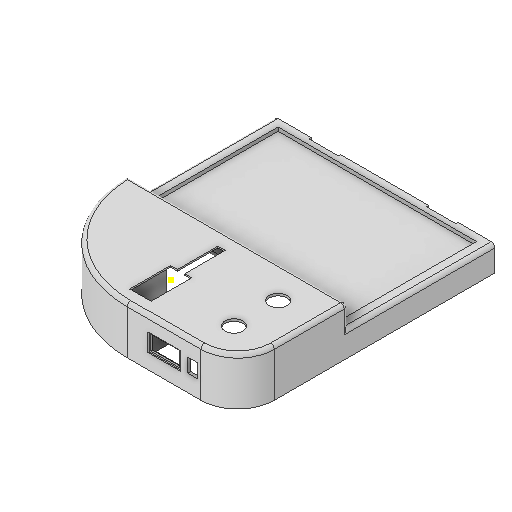
# Autodesk Inventor part: PLATE 1
Saved by Autodesk Inventor 2025.3 (Build 293356030, 356C)
## iProperties
Created: 2025-09-25
Part Number: PLATE 1
Material: 일반
Document SubType Name: Modeling
Designer: joseph
Density: 1 g/cm^3
Appearance: 기본값
Mass: 533.124 g
Surface Area: 3433.78 cm^2
Volume: 533.124 cm^3
Author: joseph
Autodesk Inventor part; units mm, degrees
ref_plane "YZ Plane" through (0, 0, 0) normal (1, 0, 0) x (0, 1, 0)
ref_plane "XZ Plane" through (0, 0, 0) normal (0, 1, 0) x (-1, 0, 0)
ref_plane "XY Plane" through (0, 0, 0) normal (0, 0, 1) x (1, 0, 0)
sketch "스케치6" plane through (0, 0, 0) normal (0, 0, 1) x (1, 0, 0)
  circle A0 centre (0, 0) radius 50
  line L0 (150, 90) -> (-150, 90)
  line L1 (-150, 90) -> (-150, 290)
  line L2 (-150, 290) -> (150, 290)
  line L3 (150, 290) -> (150, 90)
  line L4 (150, 90) -> (150, 14.5116)
  line L5 (0, -60) -> (100, -60)
  line L6 (150, 14.5116) -> (150, -10)
  arc A1 (-150, 90) -> (0, -60) centre (0, 90) ccw
  arc A2 (100, -60) -> (150, -10) centre (100, -10) ccw
  arc A3 (-147, 86) -> (17.5784, -56) centre (0, 90) ccw
  line L7 (17.5784, -56) -> (100, -56)
  arc A4 (100, -56) -> (146, -10) centre (100, -10) ccw
  line L8 (146, -10) -> (146, 14.5116)
  line L9 (146, 14.5116) -> (146, 86)
  line L10 (146, 86) -> (-147, 86)
  line L11 (-149.9467, 86) -> (-150, 86)
  point P0 (150, -60)
  point P1 (150, -60)
  point P2 (0, 290)
  dimension "d0" = 100
  dimension "d1" = 300
  dimension "d2" = 200
  dimension "d5" = 150
  dimension "d8" = 90
  dimension "d9" = 150
  dimension "d10" = 50
  dimension "d24" = 3
  constraints: 24 end point, 9 point on circle, 5 centre point, 4 parallel, 4 tangent, 3 point on line, 2 horizontal, 2 vertical, 1 coincident, 1 midpoint, 1 perpendicular, 1 vertical alignment, 2 other
  measures "d0" diameter of A0
  measures "d1" distance of L1.end L2.end
  measures "d2" distance of L0.end L1.end
  measures "d5" distance of L0.start point (150, -60)
  measures "d8" vertical distance of point (0, 0) L0.end
  measures "d9" distance of L5.start point (150, -60)
  measures "d10" radius of A2
  measures "d24" horizontal distance of L0.end L10.end
extrude "돌출1" add sketch "스케치6" against normal blind 65 contours L4 L6 A2 L5 A1 L0
extrude "돌출2" add sketch "스케치6" against normal blind 3 contours L10 L9 L8 A4 L7 A3
sketch "스케치8" plane through (-147, 86, -65) normal (0, -1, 0) x (1, 0, 0)
  line L0 (293, 62) -> (0, 62) projected
  line L1 (0, 62) -> (0, 0) projected
  line L2 (293, 0) -> (0, 0) projected
  line L3 (293, 62) -> (293, 0) projected
  line L4 (0, 0) -> (293, 0)
  line L5 (293, 0) -> (293, 27.5)
  line L6 (293, 27.5) -> (0, 27.5)
  line L7 (0, 27.5) -> (0, 0)
  point P0 (147, 65)
  dimension "d17" = 27.5
  constraints: 8 end point, 2 parallel, 1 horizontal, 1 perpendicular, 1 point on line
  measures "d17" distance of L5.end L4.end
extrude "돌출3" cut sketch "스케치8" against normal blind 60 contours L3 L2 L1 L6
sketch "스케치9" plane through (0, 0, -65) normal (0, 0, -1) x (-1, 0, 0)
  line L0 (-146, -10) -> (-146, 90) projected
  line L1 (-146, 90) -> (-150, 90) projected
  line L2 (-150, 90) -> (-150, -10) projected
  arc A0 (-150, -10) -> (-100, -60) centre (-100, -10) ccw projected
  line L3 (-100, -60) -> (0, -60) projected
  arc A1 (0, -60) -> (150, 90) centre (0, 90) ccw projected
  line L4 (150, 90) -> (147, 90) projected
  line L5 (147, 90) -> (147, 86) projected
  arc A2 (-17.5784, -56) -> (147, 86) centre (0, 90) ccw projected
  line L6 (-17.5784, -56) -> (-100, -56) projected
  arc A3 (-146, -10) -> (-100, -56) centre (-100, -10) ccw projected
  line L7 (-150, 90) -> (150, 90)
  line L8 (150, 90) -> (150, 290)
  line L9 (150, 290) -> (-150, 290)
  line L10 (-150, 290) -> (-150, 90)
  line L11 (-146, 90) -> (146, 90)
  line L12 (146, 90) -> (146, 286)
  line L13 (146, 286) -> (-146, 286)
  line L14 (-146, 286) -> (-146, 90)
  point P0 (0, 0)
  point P1 (146, 90)
  dimension "d20" = 300
  dimension "d21" = 200
  dimension "d22" = 292
  dimension "d23" = 196
  constraints: 16 end point, 4 parallel, 2 horizontal, 2 perpendicular
  measures "d20" distance of L9.end L8.end
  measures "d21" distance of L8.end L7.end
  measures "d22" distance of L13.end L12.end
  measures "d23" distance of L12.end L11.end
extrude "돌출4" add sketch "스케치9" against normal blind 34.5 contours L1 L10 L9 L8 L4 L7 L12 L13 L14
sketch "스케치10" plane through (0, 0, -30.5) normal (0, 0, 1) x (1, 0, 0)
  line L0 (150, 290) -> (-150, 290) projected
  line L1 (-150, 290) -> (-150, 90) projected
  line L2 (-146, 90) -> (-150, 90) projected
  line L3 (-146, 90) -> (-146, 286) projected
  line L4 (-146, 286) -> (146, 286) projected
  line L5 (146, 286) -> (146, 90) projected
  line L6 (150, 90) -> (146, 90) projected
  line L7 (150, 90) -> (150, 290) projected
  line L8 (-150, 90) -> (150, 90)
  point P0 (0, 0)
  point P1 (-146, 90)
  constraints: 2 end point, 1 horizontal
extrude "돌출5" add sketch "스케치10" against normal blind 7
fillet "모깎기1" radius 5 2 edges at (150, 190, -30.5) (-150, 190, -30.5)
fillet "모깎기2" radius 5 7 edges at (150, 90, -33) (150, 90, -15.25) (135.3553, -45.3553, 0) (50, -60, 0) (-106.066, -16.066, 0) (150, 40, 0) (0, 90, 0)
sketch "스케치12" plane through (0, 0, 0) normal (0, 0, 1) x (1, 0, 0)
  circle A0 centre (100, -15) radius 22.5
  circle A1 centre (100, 45) radius 22.5
  circle A2 centre (100, 45) radius 12.15
  circle A3 centre (100, -15) radius 12.15
  point P0 (0, 0)
  dimension "d33" = 45
  dimension "d34" = 45
  dimension "d35" = 15
  dimension "d36" = 100
  dimension "d37" = 60
  dimension "d38" = 24.3
  dimension "d39" = 24.3
  constraints: 4 centre point, 2 coincident, 1 vertical alignment
  measures "d33" diameter of A0
  measures "d34" diameter of A1
  measures "d35" vertical distance of A0.centre point (0, 0)
  measures "d36" horizontal distance of A0.centre point (0, 0)
  measures "d37" distance of A0.centre A1.centre
  measures "d38" diameter of A2
  measures "d39" diameter of A3
extrude "돌출6" cut sketch "스케치12" against normal through all contours A2 | A3
sketch "스케치13" plane through (0, 0, -65) normal (0, 0, -1) x (-1, 0, 0)
  line L0 (-150, 290) -> (-150, -10) projected
  arc A0 (-150, -10) -> (-100, -60) centre (-100, -10) ccw projected
  line L1 (-100, -60) -> (0, -60) projected
  arc A1 (0, -60) -> (150, 90) centre (0, 90) ccw projected
  line L2 (150, 90) -> (150, 290) projected
  line L3 (150, 290) -> (-150, 290) projected
  line L4 (-146, -10) -> (-146, 286) projected
  line L5 (-146, 286) -> (146, 286) projected
  line L6 (147, 90) -> (147, 86) projected
  arc A2 (-17.5784, -56) -> (147, 86) centre (0, 90) ccw projected
  line L7 (-17.5784, -56) -> (-100, -56) projected
  arc A3 (-146, -10) -> (-100, -56) centre (-100, -10) ccw projected
  circle A4 centre (-100, -15) radius 12.15 projected
  line L8 (-100, -36) -> (-16.3347, -36)
  arc A5 (-16.3347, -36) -> (127, 86.282) centre (0, 90) ccw
  line L9 (127, 86.282) -> (127, 266)
  line L10 (127, 266) -> (-126, 266)
  line L11 (-126, 266) -> (-126, -10)
  arc A6 (-126, -10) -> (-100, -36) centre (-100, -10) ccw
  line L12 (146, 286) -> (146, 90) projected
  line L13 (146, 90) -> (147, 90) projected
  point P0 (0, 0)
  dimension "d42" = 20
  constraints: 8 end point, 4 point on circle, 2 centre point, 5 other
  measures "d42" radial gap between concentric circles of A3 A6
extrude "돌출7" add sketch "스케치13" against normal blind 3 contours L4 L5 L12 L13 L6 A2 L7 A3
sketch "스케치15" plane through (-150, 90, -65) normal (-1, 0, 0) x (0, 0, 1)
  line L0 (29.5, 200) -> (29.5, 0) projected
  line L1 (0, 200) -> (29.5, 200) projected
  line L2 (0, 0) -> (0, 200) projected
  line L3 (29.5, 0) -> (0, 0) projected
  line L4 (9.75, 190) -> (19.75, 190)
  line L5 (19.75, 190) -> (19.75, 195)
  line L6 (19.75, 195) -> (9.75, 195)
  line L7 (9.75, 195) -> (9.75, 190)
  point P0 (65, -90)
  point P1 (14.75, 195)
  point P2 (14.75, 200)
  dimension "d45" = 10
  dimension "d46" = 5
  dimension "d47" = 5
  constraints: 8 end point, 2 midpoint, 2 parallel, 1 horizontal, 1 perpendicular, 1 vertical alignment
  measures "d45" distance of L6.end L5.end
  measures "d46" distance of L5.end L4.end
  measures "d47" distance between parallel lines of L1 L6
extrude "돌출8" cut sketch "스케치15" against normal blind 10 contours L7 L6 L5 L4
sketch "스케치16" plane through (0, 0, -30.5) normal (0, 0, 1) x (1, 0, 0)
  line L0 (-145, 90) -> (-145, 290) projected
  line L1 (145, 90) -> (-145, 90) projected
  line L2 (145, 290) -> (145, 90) projected
  line L3 (145, 290) -> (-145, 290) projected
  line L4 (-135, 280) -> (-135, 100)
  line L5 (-135, 100) -> (135, 100)
  line L6 (135, 100) -> (135, 280)
  line L7 (135, 280) -> (-135, 280)
  point P0 (0, 0)
  dimension "d50" = 10
  constraints: 8 end point, 3 other
  measures "d50" distance between parallel lines of L0 L4
extrude "돌출9" cut sketch "스케치16" against normal blind 5 contours L7 L6 L5 L4
sketch "스케치17" plane through (0, 0, 0) normal (0, 0, 1) x (1, 0, 0)
  line L0 (-25, 13.2) -> (25, 13.2)
  line L1 (25, 13.2) -> (25, -55.3)
  line L2 (25, -55.3) -> (-25, -55.3)
  line L3 (-25, -55.3) -> (-25, 13.2)
  line L4 (-20.35, 13.2) -> (20.35, 13.2)
  line L5 (20.35, 13.2) -> (20.35, -48)
  line L6 (20.35, -48) -> (-20.35, -48)
  line L7 (-20.35, -48) -> (-20.35, 13.2)
  line L8 (-14.5, 13.2) -> (14.5, 13.2)
  line L9 (14.5, 13.2) -> (14.5, -42.2)
  line L10 (14.5, -42.2) -> (-14.5, -42.2)
  line L11 (-14.5, -42.2) -> (-14.5, 13.2)
  line L12 (-25, -51.9991) -> (0, -55.3)
  point P0 (0, 0)
  point P1 (0, -48)
  point P2 (0, -42.2)
  point P3 (-14.5, 13.2)
  point P4 (0, 13.2)
  dimension "d53" = 50
  dimension "d54" = 68.5
  dimension "d55" = 13.2
  dimension "d56" = 40.7
  dimension "d57" = 61.2
  dimension "d58" = 29
  dimension "d59" = 55.4
  constraints: 26 end point, 6 parallel, 4 midpoint, 3 horizontal, 3 perpendicular, 3 point on line, 3 vertical alignment
  measures "d53" distance of L1.end L2.end
  measures "d54" distance of L0.end L1.end
  measures "d55" distance from line of point (0, 0) L0
  measures "d56" distance of L5.end L6.end
  measures "d57" distance of L4.end L5.end
  measures "d58" distance of L9.end L10.end
  measures "d59" distance of L8.end L9.end
extrude "돌출10" add sketch "스케치17" against normal blind 2 contours L0 L7 L6 L5 L1 L2 L12 L3 | L0 L11 L10 L9 L5 L6 L7
sketch "스케치18" plane through (-25, 13.2, 0) normal (0, 1, 0) x (1, 0, 0)
  line L0 (10.5, 0) -> (0, 0) projected
  line L1 (10.5, 0) -> (10.5, 2) projected
  line L2 (0, 2) -> (10.5, 2) projected
  line L3 (0, 0) -> (0, 2) projected
  line L4 (50, 0) -> (39.5, 0) projected
  line L5 (50, 0) -> (50, 2) projected
  line L6 (39.5, 2) -> (50, 2) projected
  line L7 (39.5, 0) -> (39.5, 2) projected
  line L8 (50, 2) -> (0, 2)
  line L9 (0, 2) -> (0, 52)
  line L10 (0, 52) -> (50, 52)
  line L11 (50, 52) -> (50, 2)
  line L12 (39.5, 2) -> (45.2, 2)
  line L13 (45.2, 2) -> (45.2, 36.4)
  line L14 (45.2, 36.4) -> (39.5, 36.4)
  line L15 (39.5, 36.4) -> (39.5, 2)
  line L16 (10.5, 2) -> (4.8, 2)
  line L17 (4.8, 2) -> (4.8, 36.4)
  line L18 (4.8, 36.4) -> (10.5, 36.4)
  line L19 (10.5, 36.4) -> (10.5, 2)
  line L20 (10.5, 36.4) -> (4.8, 36.4)
  line L21 (4.8, 36.4) -> (4.8, 39.7)
  line L22 (4.8, 39.7) -> (10.5, 39.7)
  line L23 (10.5, 39.7) -> (10.5, 36.4)
  line L24 (45.2, 36.4) -> (39.5, 36.4)
  line L25 (39.5, 36.4) -> (39.5, 39.7)
  line L26 (39.5, 39.7) -> (45.2, 39.7)
  line L27 (45.2, 39.7) -> (45.2, 36.4)
  line L28 (39.5, 39.7) -> (10.5, 39.7)
  line L29 (10.5, 39.7) -> (10.5, 49.7)
  line L30 (10.5, 49.7) -> (39.5, 49.7)
  line L31 (39.5, 49.7) -> (39.5, 39.7)
  point P0 (25, 0)
  point P1 (0, 2)
  dimension "d62" = 50
  dimension "d63" = 5.7
  dimension "d64" = 34.4
  dimension "d65" = 5.7
  dimension "d66" = 34.4
  dimension "d67" = 3.3
  dimension "d68" = 10
  constraints: 48 end point, 12 parallel, 6 horizontal, 6 perpendicular, 4 point on line
  measures "d62" distance of L8.end L9.end
  measures "d63" distance of L14.end L13.end
  measures "d64" distance of L13.end L12.end
  measures "d65" distance of L17.end L18.end
  measures "d66" distance of L16.end L17.end
  measures "d67" distance of L20.end L21.end
  measures "d68" distance of L28.end L29.end
extrude "돌출11" add sketch "스케치18" against normal through all contours L9 L10 L11 L6 L13 L27 L26 L31 L30 L29 L22 L21 L17 L2 | L18 L21 L22 L23 | L25 L26 L27 L14
sketch "스케치19" plane through (0, 0, 0) normal (0, 0, 1) x (1, 0, 0)
  line L0 (100, -55) -> (25, -55) projected
  arc A0 (100, -55) -> (145, -10) centre (100, -10) ccw projected
  line L1 (145, 85) -> (145, -10) projected
  line L2 (-144.9138, 85) -> (145, 85) projected
  arc A1 (-144.9138, 85) -> (-2.4258, -54.9797) centre (0, 90) ccw projected
  line L3 (-2.4258, -54.9797) -> (0, -55.3) projected
  line L4 (0, -55.3) -> (25, -55.3) projected
  line L5 (25, -55.3) -> (25, -55) projected
  arc A2 (25, -43.3013) -> (-25, -43.3013) centre (0, 0) ccw projected
  line L6 (25, -43.3013) -> (25, 13.2) projected
  line L7 (25, 13.2) -> (14.5, 13.2) projected
  line L8 (14.5, 13.2) -> (14.5, -42.2) projected
  line L9 (14.5, -42.2) -> (-14.5, -42.2) projected
  line L10 (-14.5, -42.2) -> (-14.5, 13.2) projected
  line L11 (-14.5, 13.2) -> (-25, 13.2) projected
  line L12 (-25, 13.2) -> (-25, -43.3013) projected
  circle A3 centre (100, -15) radius 12.15 projected
  circle A4 centre (100, 45) radius 12.15 projected
  line L13 (-25, 13.2) -> (25, 13.2)
  constraints: 2 end point, 1 collinear
extrude "돌출12" add sketch "스케치19" against normal blind 2 contours L6 L7 L13 L11 L12 A2
sketch "스케치20" plane through (0, 0, -3) normal (0, 0, -1) x (-1, 0, 0)
  point P0 (0, 0)
sketch "스케치21" plane through (0, 0, -3) normal (0, 0, -1) x (-1, 0, 0)
  line L0 (147, 86) -> (-146, 86) projected
  line L1 (-25, 13.2) -> (25, 13.2) projected
  line L2 (-25, 13.2) -> (27.4279, 13.2)
  line L3 (27.4279, 13.2) -> (27.4279, 86)
  line L4 (27.4279, 86) -> (-25, 86)
  line L5 (-25, 86) -> (-25, 13.2)
  point P0 (0, 0)
  point P1 (22.5721, 13.2)
  constraints: 8 end point, 2 parallel, 1 horizontal, 1 perpendicular, 1 point on line
extrude "돌출13" cut sketch "스케치21" against normal blind 1
sketch "스케치22" plane through (0, 0, 0) normal (0, 0, 1) x (1, 0, 0)
  line L0 (-14.5, 13.2) -> (14.5, 13.2) projected
  line L1 (-5, 13.2) -> (5, 13.2)
  line L2 (5, 13.2) -> (5, 68.2)
  line L3 (5, 68.2) -> (-5, 68.2)
  line L4 (-5, 68.2) -> (-5, 13.2)
  point P0 (0, 0)
  point P1 (0, 13.2)
  dimension "d75" = 10
  dimension "d76" = 55
  constraints: 8 end point, 2 midpoint, 2 parallel, 1 horizontal, 1 perpendicular, 1 point on line
  measures "d75" distance of L3.end L2.end
  measures "d76" distance of L2.end L1.end
extrude "돌출14" cut sketch "스케치22" against normal blind 3
sketch "스케치23" plane through (25, 13.2, -52) normal (0, 0, -1) x (-1, 0, 0)
  line L0 (7.4216, -69.2) -> (0, -69.2) projected
  arc A0 (7.4216, -69.2) -> (50, -68.1138) centre (25, 76.8) ccw projected
  line L1 (50, 0) -> (50, -68.1138) projected
  line L2 (0, 0) -> (50, 0) projected
  line L3 (0, 0) -> (0, -69.2) projected
  circle A1 centre (7.5, -9) radius 1.6
  circle A2 centre (7.5, -31.9) radius 1.6
  circle A3 centre (42.2, -9) radius 1.6
  circle A4 centre (42.2, -31.9) radius 1.6
  point P0 (25, -13.2)
  dimension "d79" = 3.2
  dimension "d80" = 7.5
  dimension "d81" = 9
  dimension "d84" = 22.9
  dimension "d87" = 34.7
  constraints: 4 centre point, 1 horizontal, 1 vertical, 6 other
  measures "d79" diameter of A1
  measures "d80" horizontal distance of A1.centre L2.start
  measures "d81" vertical distance of L2.start A1.centre
  measures "d84" distance of A1.centre A2.centre
  measures "d87" distance of A1.centre A3.centre
extrude "돌출15" cut sketch "스케치23" against normal blind 20 contours A1 | A2 | A3 | A4
fillet "모깎기4" radius 10 11 edges at (132.5269, -42.5269, -3) (62.5, -56, -3) (146, 38, -3) (146, 86, -20.25) (85.5, 86, -3) (146, 186, -37.5) (-0.5, 86, -37.5) (-87.214, 86, -3) (-111.1763, -6.254, -3) (-25, -15.0506, -2) (25, -15.0506, -2)
fillet "모깎기5" radius 3.5 8 edges at (132.5269, -42.5269, -62) (146, 138, -62) (58.7892, -56, -62) (-96.065, -21.3396, -62) (-146, 188, -62) (0, 286, -62) (-146.5, 90, -62) (-147, 88, -62)
sketch "스케치24" plane through (0, -60, -65) normal (0, -1, 0) x (1, 0, 0)
  line L0 (30, 42.7) -> (70, 42.7)
  line L1 (70, 42.7) -> (70, 22.3)
  line L2 (70, 22.3) -> (30, 22.3)
  line L3 (30, 22.3) -> (30, 42.7)
  line L4 (0, 65) -> (0, 0) construction
  line L5 (16.3347, 0) -> (-127, 0) projected
  line L6 (72, 44.7) -> (28, 44.7)
  line L7 (28, 44.7) -> (28, 20.3)
  line L8 (28, 20.3) -> (72, 20.3)
  line L9 (72, 20.3) -> (72, 44.7)
  line L10 (82, 23) -> (96, 23)
  line L11 (96, 23) -> (96, 42)
  line L12 (96, 42) -> (82, 42)
  line L13 (82, 42) -> (82, 23)
  point P0 (30, 32.5)
  point P1 (0, 32.5)
  point P2 (82, 32.5)
  point P3 (72, 32.5)
  dimension "d94" = 40
  dimension "d95" = 20.4
  dimension "d96" = 30
  dimension "d97" = 2
  dimension "d102" = 14
  dimension "d103" = 19
  dimension "d104" = 10
  constraints: 26 end point, 6 parallel, 4 midpoint, 3 perpendicular, 2 horizontal, 2 horizontal alignment, 1 point on line, 1 vertical, 3 other
  measures "d94" distance of L1.end L2.end
  measures "d95" distance of L0.end L1.end
  measures "d96" horizontal distance of point (0, 32.5) L0.start
  measures "d97" distance between parallel lines of L0 L6
  measures "d102" distance of L12.end L11.end
  measures "d103" distance of L11.end L10.end
  measures "d104" distance between parallel lines of L9 L13
extrude "돌출16" cut sketch "스케치24" against normal blind 1.5 contours L9 L8 L7 L6
extrude "돌출17" cut sketch "스케치24" against normal blind 4 contours L0 L1 L2 L3
extrude "돌출18" cut sketch "스케치24" against normal blind 4 contours L13 L12 L11 L10
sketch "스케치25" plane through (-150, 290, -65) normal (0, 1, 0) x (1, 0, 0)
  arc A0 (0, -29.5) -> (5, -34.5) centre (5, -29.5) ccw projected
  line L0 (295, -34.5) -> (5, -34.5) projected
  arc A1 (295, -34.5) -> (300, -29.5) centre (295, -29.5) ccw projected
  line L1 (300, 0) -> (300, -29.5) projected
  line L2 (0, 0) -> (300, 0) projected
  line L3 (0, 0) -> (0, -29.5) projected
  line L4 (250, -34.5) -> (210, -34.5)
  line L5 (210, -34.5) -> (210, -18.5)
  line L6 (210, -18.5) -> (250, -18.5)
  line L7 (250, -18.5) -> (250, -34.5)
  line L8 (90, -34.5) -> (50, -34.5)
  line L9 (50, -34.5) -> (50, -18.5)
  line L10 (50, -18.5) -> (90, -18.5)
  line L11 (90, -18.5) -> (90, -34.5)
  point P0 (150, -65)
  dimension "d107" = 40
  dimension "d108" = 16
  dimension "d109" = 40
  dimension "d110" = 16
  dimension "d111" = 50
  dimension "d112" = 50
  constraints: 16 end point, 4 parallel, 2 horizontal, 2 perpendicular, 2 point on line
  measures "d107" distance of L5.end L6.end
  measures "d108" distance of L4.end L5.end
  measures "d109" distance of L9.end L10.end
  measures "d110" distance of L8.end L9.end
  measures "d111" distance from line of L1.start L7
  measures "d112" distance from line of L3 L9.end
extrude "돌출19" cut sketch "스케치25" against normal blind 1 contours L9 L10 L11 L0 | L5 L6 L7 L0
fillet "모깎기6" radius 2 2 edges at (-80, 289, -30.5) (80, 289, -30.5) inverted yes
